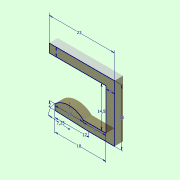
# Autodesk Inventor part: Cuvette_retainer
Saved by Autodesk Inventor 2015 (Build 190159000, 159)
## iProperties
Created: 2015-05-25
Part Number: Cuvette_retainer
Material: Generic
Document SubType Name: Modeling
Designer: Openlab
Density: 1 g/cm^3
Appearance: Polycarbonate - Smoked
Author: Openlab
Autodesk Inventor part; units mm, degrees
ref_plane "YZ Plane" through (0, 0, 0) normal (1, 0, 0) x (0, 1, 0)
ref_plane "XZ Plane" through (0, 0, 0) normal (0, 1, 0) x (-1, 0, 0)
ref_plane "XY Plane" through (0, 0, 0) normal (0, 0, 1) x (1, 0, 0)
sketch "Sketch1" plane through (0, 0, 0) normal (0, 1, 0) x (-1, 0, 0)
  line L0 (0, 0) -> (23, 0)
  line L1 (23, 0) -> (23, -3)
  line L2 (0, 0) -> (0, -20)
  line L3 (0, -20) -> (9, -20)
  line L4 (21, -19.5) -> (21, -17.5)
  line L5 (11, -17.5) -> (3, -17.5)
  line L6 (3, -17.5) -> (3, -3)
  line L7 (3, -3) -> (23, -3)
  arc A0 (21, -17.5) -> (11, -17.5) centre (16, -22.75) ccw
  line L8 (9, -20) -> (21, -19.5)
  point P0 (16, -15.5)
  dimension "d1" = 3
  dimension "d2" = 20
  dimension "d3" = 3
  dimension "d4" = 23
  dimension "d9" = 12
  dimension "d10" = 2
  dimension "d11" = 10
  dimension "d12" = 8
  dimension "d13" = 14.5
  dimension "d14" = 7.25
  dimension "d15" = 18
  constraints: 18 end point, 4 perpendicular, 3 point on circle, 2 vertical, 1 centre point, 1 horizontal
  measures "d1" distance of L0.end L1.end
  measures "d2" distance of L0.start L2.end
  measures "d3" distance between parallel lines of L2 L6
  measures "d4" distance of L0.start L0.end
  measures "d9" horizontal distance of L3.end L4.start
  measures "d10" distance of L4.start L4.end
  measures "d11" distance of L5.start L4.end
  measures "d12" distance of L5.start L5.end
  measures "d13" distance of L5.end L6.end
  measures "d14" radius of A0
  measures "d15" distance between parallel lines of L6 L4
extrude "Extrusion1" add sketch "Sketch1" along normal blind 3
body "Solid1"
